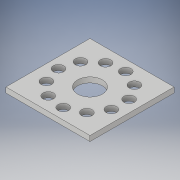
# Autodesk Inventor part: basePlate
Saved by Autodesk Inventor 2019 (Build 230136000, 136)
## iProperties
Created: 2019-05-17
Part Number: basePlate
Material: Generic
Document SubType Name: Modeling
Designer: Alex Jones
Density: 1 g/cm^3
Appearance: Default
Author: Alex Jones
Autodesk Inventor part; units mm, degrees
ref_plane "YZ Plane" through (0, 0, 0) normal (1, 0, 0) x (0, 1, 0)
ref_plane "XZ Plane" through (0, 0, 0) normal (0, 1, 0) x (-1, 0, 0)
ref_plane "XY Plane" through (0, 0, 0) normal (0, 0, 1) x (1, 0, 0)
sketch "Sketch1" plane through (0, 0, 0) normal (0, 1, 0) x (-1, 0, 0)
  circle A0 centre (0, 0) radius 19.05 construction
  circle A1 centre (19.05, 0) radius 3.175
  circle A2 centre (16.0259, 10.2992) radius 3.175
  circle A3 centre (7.9137, 17.3285) radius 3.175
  circle A4 centre (-2.7111, 18.8561) radius 3.175
  circle A5 centre (-12.4751, 14.397) radius 3.175
  circle A6 centre (-18.2783, 5.367) radius 3.175
  circle A7 centre (-18.2783, -5.367) radius 3.175
  circle A8 centre (-12.4751, -14.397) radius 3.175
  circle A9 centre (-2.7111, -18.8561) radius 3.175
  circle A10 centre (7.9137, -17.3285) radius 3.175
  circle A11 centre (16.0259, -10.2992) radius 3.175
  line L0 (-25.4, 25.4) -> (25.4, 25.4)
  line L1 (25.4, 25.4) -> (25.4, -25.4)
  line L2 (25.4, -25.4) -> (-25.4, -25.4)
  line L3 (-25.4, -25.4) -> (-25.4, 25.4)
  line L4 (-25.4, 25.4) -> (25.4, -25.4) construction
  line L5 (25.4, 25.4) -> (-25.4, -25.4) construction
  dimension "d0" = 38.1
  dimension "d1" = 6.35
  dimension "d4" = 360
  dimension "d6" = 50.8
  dimension "d7" = 50.8
  constraints: 12 end point, 11 centre point, 2 midpoint, 2 parallel, 1 coincident, 1 horizontal, 1 horizontal alignment, 1 perpendicular, 25 other
  measures "d1" diameter of A1
  measures "d6" distance of L1.end L2.end
  measures "d7" distance of L0.end L1.end
extrude "Extrusion1" add sketch "Sketch1" along normal blind 3.175
sketch "Sketch2" plane through (0, 3.175, 0) normal (0, 1, 0) x (1, 0, 0)
  circle A0 centre (0, 0) radius 7.5
  dimension "d10" = 15
  constraints: 1 centre point, 1 coincident
  measures "d10" diameter of A0
extrude "Extrusion2" cut sketch "Sketch2" against normal blind 3.175
body "Solid1"
